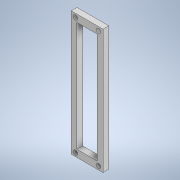
# Autodesk Inventor part: PartC
Saved by Autodesk Inventor 2020.2 (Build 242310000, 310)
## iProperties
Created: 2020-12-02
Part Number: PartC
Material: Generic
Document SubType Name: Modeling
Designer: Acer
Density: 1 g/cm^3
Appearance: Default
Author: Acer
Autodesk Inventor part; units mm, degrees
ref_plane "YZ Plane" through (0, 0, 0) normal (1, 0, 0) x (0, 1, 0)
ref_plane "XZ Plane" through (0, 0, 0) normal (0, 1, 0) x (-1, 0, 0)
ref_plane "XY Plane" through (0, 0, 0) normal (0, 0, 1) x (1, 0, 0)
sketch "Sketch1" plane through (0, 0, 0) normal (0, 0, 1) x (1, 0, 0)
  line L0 (-11, 43) -> (11, 43)
  line L1 (11, 43) -> (11, -43)
  line L2 (11, -43) -> (-11, -43)
  line L3 (-11, -43) -> (-11, 43)
  line L4 (-11, 43) -> (11, -43) construction
  line L5 (11, 43) -> (-11, -43) construction
  circle A0 centre (-8, 40.5) radius 1.5
  circle A1 centre (8, 40.5) radius 1.5
  circle A2 centre (-8, -40.5) radius 1.5
  circle A3 centre (8, -40.5) radius 1.5
  line L6 (7, 38) -> (-7, 38)
  line L7 (-7, 38) -> (-7, -38)
  line L8 (-7, -38) -> (7, -38)
  line L9 (7, -38) -> (7, 38)
  line L10 (7, 38) -> (-7, -38) construction
  line L11 (-7, 38) -> (7, -38) construction
  point P0 (0, 0)
  dimension "d0" = 22
  dimension "d1" = 86
  dimension "d2" = 3
  dimension "d3" = 3
  dimension "d4" = 3
  dimension "d5" = 3
  dimension "d6" = 3
  dimension "d7" = 2.5
  dimension "d8" = 3
  dimension "d9" = 2.5
  dimension "d10" = 2.5
  dimension "d11" = 3
  dimension "d12" = 3
  dimension "d13" = 2.5
  dimension "d14" = 14
  dimension "d15" = 76
  constraints: 24 end point, 4 centre point, 4 midpoint, 4 parallel, 2 horizontal, 2 perpendicular
  measures "d0" distance of L1.end L2.end
  measures "d1" distance of L0.end L1.end
  measures "d2" diameter of A0
  measures "d3" diameter of A1
  measures "d4" diameter of A2
  measures "d5" diameter of A3
  measures "d6" distance from line of L3 A0.centre
  measures "d7" distance from line of L0 A0.centre
  measures "d8" distance from line of L1 A1.centre
  measures "d9" distance from line of L0 A1.centre
  measures "d10" distance from line of L2 A2.centre
  measures "d11" distance from line of L3 A2.centre
  measures "d12" distance from line of L1 A3.centre
  measures "d13" distance from line of L2 A3.centre
  measures "d14" distance of L8.end L7.end
  measures "d15" distance of L7.end L6.end
extrude "Extrusion1" add sketch "Sketch1" along normal blind 4
body "Solid1"
